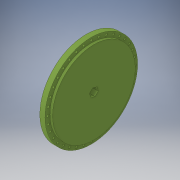
# Autodesk Inventor part: wheel hub
Saved by Autodesk Inventor 2018 (Build 220112000, 112)
## iProperties
Created: 2018-03-08
Part Number: wheel hub
Material: Generic
Document SubType Name: Modeling
Designer: prakh
Density: 1 g/cm^3
Appearance: Olive Green
Author: prakh
Autodesk Inventor part; units mm, degrees
ref_plane "YZ Plane" through (0, 0, 0) normal (1, 0, 0) x (0, 1, 0)
ref_plane "XZ Plane" through (0, 0, 0) normal (0, 1, 0) x (-1, 0, 0)
ref_plane "XY Plane" through (0, 0, 0) normal (0, 0, 1) x (1, 0, 0)
sketch "Sketch1" plane through (0, 0, 0) normal (1, 0, 0) x (0, 1, 0)
  circle A0 centre (0, 0) radius 57.15
  line L0 (5.3769, 1.4637) -> (3.9561, -3.9247)
  line L1 (3.9561, -3.9247) -> (-1.4208, -5.3884)
  line L2 (-1.4208, -5.3884) -> (-5.3769, -1.4637)
  line L3 (-5.3769, -1.4637) -> (-3.9561, 3.9247)
  line L4 (-3.9561, 3.9247) -> (1.4208, 5.3884)
  line L5 (1.4208, 5.3884) -> (5.3769, 1.4637)
  dimension "d0" = 114.3
  dimension "d1" = 9.652
  constraints: 12 end point, 2 coincident, 1 centre point, 13 other
  measures "d0" diameter of A0
  measures "d1" distance between parallel lines of L3 L0
extrude "Extrusion1" add sketch "Sketch1" along normal blind 6.35
sketch "Sketch2" plane through (6.35, 0, 0) normal (1, 0, 0) x (0, 0, -1)
  circle A0 centre (0, 0) radius 50.9905
  line L0 (3.9247, 3.9561) -> (5.3884, -1.4208) projected
  line L1 (5.3884, -1.4208) -> (1.4637, -5.3769) projected
  line L2 (1.4637, -5.3769) -> (-3.9247, -3.9561) projected
  line L3 (-3.9247, -3.9561) -> (-5.3884, 1.4208) projected
  line L4 (-5.3884, 1.4208) -> (-1.4637, 5.3769) projected
  line L5 (-1.4637, 5.3769) -> (3.9247, 3.9561) projected
  circle A1 centre (0, 0) radius 57.15 projected
  dimension "d4" = 101.981
  constraints: 1 centre point, 1 coincident
  measures "d4" diameter of A0
extrude "Extrusion2" add sketch "Sketch2" along normal blind 3.175 contours A0
sketch "Sketch3" plane through (0, 0, 0) normal (-1, 0, 0) x (0, 0, 1)
  circle A0 centre (0, 53.975) radius 1.397
  point P0 (0, 0)
  dimension "d7" = 2.794
  dimension "d8" = 53.975
  constraints: 1 centre point, 1 vertical alignment
  measures "d7" diameter of A0
  measures "d8" distance of A0.centre point (0, 0)
extrude "Extrusion3" cut sketch "Sketch3" against normal blind 6.35
pattern_circular "Circular Pattern1" count 36 over 360 about axis through (-10, 0, 0) along (1, 0, 0) of "Extrusion3"
body "Solid1"
